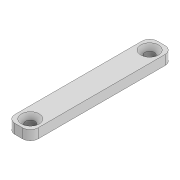
# Autodesk Inventor part: кронштейн wemos
Saved by Autodesk Inventor 2021 (Build 250183000, 183)
## iProperties
Created: 2023-02-17
Part Number: кронштейн wemos
Material: Типовые
Document SubType Name: Modeling
Designer: Tasya
Density: 1 g/cm^3
Appearance: По умолчанию
Author: Tasya
Autodesk Inventor part; units mm, degrees
ref_plane "YZ Plane" through (0, 0, 0) normal (1, 0, 0) x (0, 1, 0)
ref_plane "XZ Plane" through (0, 0, 0) normal (0, 1, 0) x (-1, 0, 0)
ref_plane "XY Plane" through (0, 0, 0) normal (0, 0, 1) x (1, 0, 0)
sketch "Эскиз1" plane through (0, 0, 0) normal (0, 1, 0) x (-1, 0, 0)
  line L0 (-1, 18.5) -> (1, 18.5)
  line L1 (3, 16.5) -> (3, -16.5)
  line L2 (1, -18.5) -> (-1, -18.5)
  line L3 (-3, -16.5) -> (-3, 16.5)
  line L4 (-3, 18.5) -> (3, -18.5) construction
  line L5 (3, 18.5) -> (-3, -18.5) construction
  arc A0 (3, 16.5) -> (1, 18.5) centre (1, 16.5) ccw
  arc A1 (-1, 18.5) -> (-3, 16.5) centre (-1, 16.5) ccw
  arc A2 (1, -18.5) -> (3, -16.5) centre (1, -16.5) ccw
  arc A3 (-3, -16.5) -> (-1, -18.5) centre (-1, -16.5) ccw
  circle A4 centre (0, 15.5) radius 2.3
  line L6 (0, 0) -> (0, 8.5528) construction
  line L7 (3, 0) -> (-3, 0) construction
  circle A5 centre (0, -15.5) radius 2.3
  dimension "d0" = 6
  dimension "d1" = 2
  dimension "d2" = 2
  dimension "d3" = 4.6
  dimension "d4" = 3
  dimension "d5" = 15.5
  constraints: 16 end point, 9 point on line, 8 point on circle, 8 tangent, 6 centre point, 4 midpoint, 2 equal radius, 2 parallel, 1 horizontal, 1 perpendicular, 1 symmetric about line, 1 vertical, 1 other
  measures "d0" distance of L4.end L5.end
  measures "d1" radius of A0
  measures "d2" radius of A1
  measures "d3" diameter of A4
  measures "d4" distance from line of A4.centre L0
  measures "d5" distance of L6.start A4.centre
extrude "Выдавливание1" add sketch "Эскиз1" along normal blind 2.5 contours L0 A0 L1 A2 L2 A3 L3 A1 | A4 | A5
sketch "Эскиз2" plane through (0, 2.5, 0) normal (0, 1, 0) x (1, 0, 0)
  circle A0 centre (0, -15.5) radius 2.3 projected
  circle A1 centre (0, 15.5) radius 2.3 projected
  point P0 (0, 0)
hole "Отверстие1" at (0, 2.5, 15.5) at (0, 2.5, -15.5) direction (0, -1, 0) diameter 2.4 depth 4 countersink diameter 4.6 countersink angle 90 clearance for "с потайной головкой ГОСТ 12876-67" size "M2" standard "ГОСТ"
